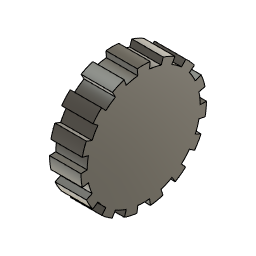
Wheels old (1) (Autodesk Fusion 360 design; units mm, degrees)
Autodesk Fusion 360 part; units mm, degrees
note: some values were not read from the file. Chosen so that the rebuilt part matches the saved one: which face or edge a step refers to.
sketch "Sketch1" plane through (0, 0, 0) normal (1, 0, 0) x (0, 1, 0)
  line L0 (107.0073, 34.7229) -> (118.8971, 38.581)
  line L1 (97.4397, 56.2295) -> (108.2663, 62.4772)
  line L2 (83.5399, 75.3481) -> (92.8221, 83.7201)
  line L3 (66.1554, 90.9929) -> (73.5061, 101.1032)
  line L4 (45.8349, 102.7395) -> (50.9277, 114.155)
  line L5 (0, 112.5) -> (0, 125)
  line L6 (23.3418, 110.0518) -> (25.9354, 122.2798)
  line L7 (0, 112.5) -> (0, 125)
  line L8 (-45.8349, 102.7395) -> (-50.9277, 114.155)
  line L9 (-23.3418, 110.0518) -> (-25.9354, 122.2798)
  line L10 (-66.1554, 90.9929) -> (-73.5061, 101.1032)
  line L11 (-83.5399, 75.3481) -> (-92.8221, 83.7201)
  line L12 (-97.4397, 56.2295) -> (-108.2663, 62.4772)
  line L13 (-107.0073, 34.7229) -> (-118.8971, 38.581)
  line L14 (111.8775, 11.818) -> (124.3084, 13.1312)
  line L15 (-111.8775, 11.818) -> (-124.3084, 13.1312)
  line L16 (111.8775, -11.818) -> (124.3084, -13.1312)
  line L17 (107.0073, -34.7229) -> (118.8971, -38.581)
  line L18 (97.4397, -56.2295) -> (108.2663, -62.4772)
  line L19 (83.5399, -75.3481) -> (92.8221, -83.7201)
  line L20 (66.1554, -90.9929) -> (73.5061, -101.1032)
  line L21 (45.8349, -102.7395) -> (50.9277, -114.155)
  line L22 (23.3418, -110.0518) -> (25.9354, -122.2798)
  line L23 (0, -112.5) -> (0, -125)
  line L24 (-111.8775, -11.818) -> (-124.3084, -13.1312)
  line L25 (-107.0073, -34.7229) -> (-118.8971, -38.581)
  line L26 (-97.4397, -56.2295) -> (-108.2663, -62.4772)
  line L27 (-83.5399, -75.3481) -> (-92.8221, -83.7201)
  line L28 (-66.1554, -90.9929) -> (-73.5061, -101.1032)
  line L29 (-45.8349, -102.7395) -> (-50.9277, -114.155)
  line L30 (-23.3418, -110.0518) -> (-25.9354, -122.2798)
  arc A0 (50.9277, 114.155) -> (25.9354, 122.2798) centre (0, 0) ccw
  arc A1 (92.8221, 83.7201) -> (73.5061, 101.1032) centre (0, 0) ccw
  arc A2 (118.8971, 38.581) -> (108.2663, 62.4772) centre (0, 0) ccw
  arc A3 (124.3084, -13.1312) -> (124.3084, 13.1312) centre (0, 0) ccw
  arc A4 (108.2663, -62.4772) -> (118.8971, -38.581) centre (0, 0) ccw
  arc A5 (73.5061, -101.1032) -> (92.8221, -83.7201) centre (0, 0) ccw
  arc A6 (25.9354, -122.2798) -> (50.9277, -114.155) centre (0, 0) ccw
  arc A7 (-25.9354, -122.2798) -> (0, -125) centre (0, 0) ccw
  arc A8 (-73.5061, -101.1032) -> (-50.9277, -114.155) centre (0, 0) ccw
  arc A9 (-108.2663, -62.4772) -> (-92.8221, -83.7201) centre (0, 0) ccw
  arc A10 (-124.3084, -13.1312) -> (-118.8971, -38.581) centre (0, 0) ccw
  arc A11 (-118.8971, 38.581) -> (-124.3084, 13.1312) centre (0, 0) ccw
  arc A12 (-92.8221, 83.7201) -> (-108.2663, 62.4772) centre (0, 0) ccw
  arc A13 (0, 125) -> (-25.9354, 122.2798) centre (0, 0) ccw
  arc A14 (-50.9277, 114.155) -> (-73.5061, 101.1032) centre (0, 0) ccw
  arc A15 (-23.3418, 110.0518) -> (-45.8349, 102.7395) centre (0, 0) ccw
  arc A16 (-66.1554, 90.9929) -> (-83.5399, 75.3481) centre (0, 0) ccw
  arc A17 (-97.4397, 56.2295) -> (-107.0073, 34.7229) centre (0, 0) ccw
  arc A18 (-111.8775, 11.818) -> (-111.8775, -11.818) centre (0, 0) ccw
  arc A19 (-107.0073, -34.7229) -> (-97.4397, -56.2295) centre (0, 0) ccw
  arc A20 (-83.5399, -75.3481) -> (-66.1554, -90.9929) centre (0, 0) ccw
  arc A21 (-45.8349, -102.7395) -> (-23.3418, -110.0518) centre (0, 0) ccw
  arc A22 (0, -112.5) -> (23.3418, -110.0518) centre (0, 0) ccw
  arc A23 (45.8349, -102.7395) -> (66.1554, -90.9929) centre (0, 0) ccw
  arc A24 (83.5399, -75.3481) -> (97.4397, -56.2295) centre (0, 0) ccw
  arc A25 (107.0073, -34.7229) -> (111.8775, -11.818) centre (0, 0) ccw
  arc A26 (111.8775, 11.818) -> (107.0073, 34.7229) centre (0, 0) ccw
  arc A27 (97.4397, 56.2295) -> (83.5399, 75.3481) centre (0, 0) ccw
  arc A28 (66.1554, 90.9929) -> (45.8349, 102.7395) centre (0, 0) ccw
  arc A29 (23.3418, 110.0518) -> (0, 112.5) centre (0, 0) ccw
  dimension "d3" = 250
  dimension "d4" = 225
  dimension "d5" = 12.4308
  constraint coincident A0.centre A1.centre
  constraint coincident L0.end A13
  constraint coincident L2.end A13
  constraint coincident L4.end A13
  constraint symmetric L0.end L5 L13.end
  constraint symmetric L2.end L5 L11.end
  constraint symmetric L3.end L5 L10.end
  constraint symmetric L4.end L5 L8.end
  constraint coincident L10.start A15
  constraint coincident L11.start A15
  constraint coincident L12.start A15
  constraint coincident L13.start A15
  constraint coincident L15.start A15
  constraint coincident L24.start A15
  constraint coincident L25.start A15
  constraint coincident L27.start A15
  constraint coincident L28.start A15
  constraint coincident L29.start A15
  constraint coincident L30.start A15
  constraint coincident L23.start A15
  constraint coincident L22.start A15
  constraint coincident L21.start A15
  constraint coincident L20.start A15
  constraint coincident L19.start A15
  constraint coincident L18.start A15
  constraint coincident L17.start A15
  constraint coincident L16.start A15
  constraint coincident L14.start A15
  constraint coincident L0.start A15
  constraint coincident L1.start A15
  constraint coincident L2.start A15
  constraint coincident L3.start A15
  constraint coincident L4.start A15
  constraint coincident L6.start A15
  constraint coincident L26.start A15
  constraint coincident L16.end A13
  constraint coincident L18.end A13
  constraint coincident L30.end A13
  constraint coincident L22.end A13
  constraint coincident L26.end A13
  constraint coincident L24.end A13
  constraint concentric A0 A13
  constraint concentric A1 A13
  constraint concentric A2 A13
  constraint concentric A3 A13
  constraint concentric A4 A13
  constraint concentric A5 A13
  constraint concentric A6 A13
  constraint concentric A7 A13
  constraint concentric A8 A13
  constraint concentric A9 A13
  constraint concentric A10 A13
  constraint concentric A11 A13
  constraint concentric A12 A13
  constraint concentric A13 A14
  constraint concentric A15 A16
  constraint concentric A16 A17
  constraint concentric A17 A18
  constraint concentric A18 A19
  constraint concentric A19 A20
  constraint concentric A20 A21
  constraint concentric A21 A22
  constraint concentric A22 A23
  constraint concentric A23 A24
  constraint concentric A24 A25
  constraint concentric A25 A26
  constraint concentric A26 A27
  constraint concentric A27 A28
  constraint concentric A28 A29
  measures "d3" diameter of A13
  measures "d4" diameter of A15
  measures "d5" horizontal distance of L14.start L14.end
extrude "Extrude1" add sketch "Sketch1" along normal blind 20
extrude "Extrude2" cut 1 faces at (0, 4.7652, -44.9254) along direction (1, 0, 0) blind 20
sketch "Sketch4" plane through (0, 0, 0) normal (1, 0, 0) x (0, 1, 0)
sketch "Sketch5" plane through (0, 0, 0) normal (1, 0, 0) x (0, 1, 0)
sketch "Sketch6" plane through (0, 0, 0) normal (1, 0, 0) x (0, 1, 0)
sketch "Sketch7" plane through (0, 0, 0) normal (1, 0, 0) x (0, 1, 0)
sketch "Sketch8" plane through (0, 0, 0) normal (1, 0, 0) x (0, 1, 0)
sketch "Sketch9" plane through (0, 0, 0) normal (1, 0, 0) x (0, 1, 0)
sketch "Sketch10" plane through (0, 0, 0) normal (1, 0, 0) x (0, 1, 0)
sketch "Sketch11" plane through (0, 0, 0) normal (1, 0, 0) x (0, 1, 0)
  circle A0 centre (0, 0) radius 90
  circle A1 centre (0, 0) radius 100
  line L0 (90, 0) -> (99.9996, 0.2793)
  line L1 (90, 0) -> (99.9996, -0.2793)
  line L2 (82.2191, -36.6063) -> (91.2406, -40.9287)
  line L3 (82.2191, -36.6063) -> (91.4678, -40.4183)
  line L4 (27.8115, -85.5951) -> (30.6359, -95.1916)
  line L5 (27.8115, -85.5951) -> (31.1672, -95.019)
  line L6 (60.2218, -66.883) -> (67.1204, -74.1273)
  line L7 (60.2218, -66.883) -> (66.7052, -74.5011)
  line L8 (-88.0333, -18.7121) -> (-97.8725, -20.5179)
  line L9 (-88.0333, -18.7121) -> (-97.7563, -21.0643)
  line L10 (-72.8115, -52.9007) -> (-81.0656, -58.5523)
  line L11 (-72.8115, -52.9007) -> (-80.7372, -59.0043)
  line L12 (-45, -77.9423) -> (-50.2417, -86.4625)
  line L13 (-45, -77.9423) -> (-49.7579, -86.7419)
  line L14 (-9.4076, -89.507) -> (-10.7306, -99.4226)
  line L15 (-9.4076, -89.507) -> (-10.175, -99.481)
  line L16 (-88.0333, 18.7121) -> (-97.8725, 20.5179)
  line L17 (-88.0333, 18.7121) -> (-97.7563, 21.0643)
  line L18 (-72.8115, 52.9007) -> (-81.0656, 58.5523)
  line L19 (-72.8115, 52.9007) -> (-80.7372, 59.0043)
  line L20 (-45, 77.9423) -> (-49.7579, 86.7419)
  line L21 (-45, 77.9423) -> (-50.2417, 86.4625)
  line L22 (-9.4076, 89.507) -> (-10.7306, 99.4226)
  line L23 (-9.4076, 89.507) -> (-10.175, 99.481)
  line L24 (27.8115, 85.5951) -> (30.6359, 95.1916)
  line L25 (27.8115, 85.5951) -> (31.1672, 95.019)
  line L26 (60.2218, 66.883) -> (66.7052, 74.5011)
  line L27 (60.2218, 66.883) -> (67.1204, 74.1273)
  line L28 (82.2191, 36.6063) -> (91.4678, 40.4183)
  line L29 (82.2191, 36.6063) -> (91.2406, 40.9287)
  line L30 (90, 0) -> (99.9996, -0.2793)
  line L31 (90, 0) -> (99.9996, 0.2793)
  line L32 (88.0333, -18.7121) -> (97.8725, -20.5179)
  line L33 (9.4076, 89.507) -> (10.7306, 99.4226)
  line L34 (72.8115, 52.9007) -> (80.7372, 59.0043)
  line L35 (9.4076, 89.507) -> (10.175, 99.481)
  line L36 (45, 77.9423) -> (50.2417, 86.4625)
  line L37 (88.0333, 18.7121) -> (97.8725, 20.5179)
  circle A2 centre (0, 0) radius 100
  line L38 (-90, 0) -> (-99.9996, 0.2793)
  line L39 (9.4076, -89.507) -> (10.175, -99.481)
  line L40 (72.8115, 52.9007) -> (81.0656, 58.5523)
  line L41 (45, 77.9423) -> (49.7579, 86.7419)
  line L42 (-60.2218, -66.883) -> (-66.7052, -74.5011)
  line L43 (-82.2191, -36.6063) -> (-91.4678, -40.4183)
  line L44 (88.0333, 18.7121) -> (97.7563, 21.0643)
  line L45 (45, -77.9423) -> (49.7579, -86.7419)
  circle A3 centre (0, 0) radius 90
  line L46 (72.8115, -52.9007) -> (80.7372, -59.0043)
  line L47 (88.0333, 18.7121) -> (97.7563, 21.0643)
  line L48 (72.8115, -52.9007) -> (81.0656, -58.5523)
  line L49 (45, -77.9423) -> (50.2417, -86.4625)
  line L50 (88.0333, 18.7121) -> (97.8725, 20.5179)
  line L51 (88.0333, -18.7121) -> (97.7563, -21.0643)
  line L52 (-27.8115, 85.5951) -> (-31.1672, 95.019)
  line L53 (9.4076, -89.507) -> (10.7306, -99.4226)
  line L54 (-60.2218, 66.883) -> (-66.7052, 74.5011)
  line L55 (-82.2191, 36.6063) -> (-91.4678, 40.4183)
  line L56 (-27.8115, 85.5951) -> (-30.6359, 95.1916)
  line L57 (-60.2218, -66.883) -> (-67.1204, -74.1273)
  line L58 (-27.8115, -85.5951) -> (-30.6359, -95.1916)
  line L59 (-60.2218, 66.883) -> (-67.1204, 74.1273)
  line L60 (-82.2191, -36.6063) -> (-91.2406, -40.9287)
  line L61 (-27.8115, -85.5951) -> (-31.1672, -95.019)
  line L62 (-82.2191, 36.6063) -> (-91.2406, 40.9287)
  line L63 (-90, 0) -> (-99.9996, -0.2793)
  line L64 (527.8115, 85.5951) -> (530.6359, 95.1916)
  line L65 (410, 0) -> (400.0004, -0.2793)
  line L66 (560.2218, 66.883) -> (566.7052, 74.5011)
  line L67 (582.2191, 36.6063) -> (591.2406, 40.9287)
  line L68 (588.0333, -18.7121) -> (597.7563, -21.0643)
  line L69 (582.2191, 36.6063) -> (591.4678, 40.4183)
  line L70 (588.0333, -18.7121) -> (597.8725, -20.5179)
  line L71 (545, 77.9423) -> (549.7579, 86.7419)
  line L72 (490.5924, 89.507) -> (489.825, 99.481)
  line L73 (411.9667, 18.7121) -> (402.2437, 21.0643)
  line L74 (455, 77.9423) -> (450.2421, 86.7419)
  line L75 (545, -77.9423) -> (549.7579, -86.7419)
  line L76 (527.8115, -85.5951) -> (530.6359, -95.1916)
  line L77 (417.7809, 36.6063) -> (408.5322, 40.4183)
  line L78 (590, 0) -> (599.9996, 0.2793)
  line L79 (545, -77.9423) -> (550.2417, -86.4625)
  line L80 (590, 0) -> (599.9996, -0.2793)
  line L81 (417.7809, 36.6063) -> (408.7594, 40.9287)
  line L82 (590, 0) -> (599.9996, -0.2793)
  line L83 (411.9667, 18.7121) -> (402.1275, 20.5179)
  line L84 (588.0333, 18.7121) -> (597.7563, 21.0643)
  line L85 (527.8115, 85.5951) -> (531.1672, 95.019)
  line L86 (545, 77.9423) -> (550.2417, 86.4625)
  line L87 (509.4076, 89.507) -> (510.7306, 99.4226)
  line L88 (572.8115, 52.9007) -> (580.7372, 59.0043)
  line L89 (560.2218, 66.883) -> (567.1204, 74.1273)
  line L90 (588.0333, 18.7121) -> (597.7563, 21.0643)
  line L91 (582.2191, -36.6063) -> (591.4678, -40.4183)
  line L92 (427.1885, 52.9007) -> (419.2628, 59.0043)
  line L93 (439.7782, 66.883) -> (433.2948, 74.5011)
  line L94 (572.8115, -52.9007) -> (581.0656, -58.5523)
  line L95 (417.7809, -36.6063) -> (408.7594, -40.9287)
  line L96 (472.1885, 85.5951) -> (468.8328, 95.019)
  line L97 (560.2218, -66.883) -> (567.1204, -74.1273)
  line L98 (590, 0) -> (599.9996, 0.2793)
  line L99 (527.8115, -85.5951) -> (531.1672, -95.019)
  line L100 (509.4076, -89.507) -> (510.175, -99.481)
  line L101 (427.1885, -52.9007) -> (419.2628, -59.0043)
  line L102 (472.1885, -85.5951) -> (469.3641, -95.1916)
  line L103 (582.2191, -36.6063) -> (591.2406, -40.9287)
  line L104 (490.5924, -89.507) -> (489.2694, -99.4226)
  line L105 (509.4076, -89.507) -> (510.7306, -99.4226)
  line L106 (490.5924, 89.507) -> (489.2694, 99.4226)
  line L107 (472.1885, -85.5951) -> (468.8328, -95.019)
  line L108 (439.7782, 66.883) -> (432.8796, 74.1273)
  line L109 (572.8115, -52.9007) -> (580.7372, -59.0043)
  line L110 (472.1885, 85.5951) -> (469.3641, 95.1916)
  line L111 (455, 77.9423) -> (449.7583, 86.4625)
  line L112 (572.8115, 52.9007) -> (581.0656, 58.5523)
  line L113 (560.2218, -66.883) -> (566.7052, -74.5011)
  line L114 (410, 0) -> (400.0004, 0.2793)
  line L115 (455, -77.9423) -> (449.7583, -86.4625)
  line L116 (439.7782, -66.883) -> (432.8796, -74.1273)
  line L117 (417.7809, -36.6063) -> (408.5322, -40.4183)
  line L118 (455, -77.9423) -> (450.2421, -86.7419)
  line L119 (509.4076, 89.507) -> (510.175, 99.481)
  line L120 (411.9667, -18.7121) -> (402.1275, -20.5179)
  line L121 (427.1885, 52.9007) -> (418.9344, 58.5523)
  line L122 (490.5924, -89.507) -> (489.825, -99.481)
  line L123 (411.9667, -18.7121) -> (402.2437, -21.0643)
  line L124 (427.1885, -52.9007) -> (418.9344, -58.5523)
  line L125 (439.7782, -66.883) -> (433.2948, -74.5011)
  line L126 (0, 900) -> (500, 900)
  line L127 (0, 900) -> (0, 800)
  arc A4 (0, 900) -> (0, 700) centre (0, 800) ccw
  line L128 (0, 700) -> (500, 700)
  arc A5 (500, 700) -> (500, 900) centre (500, 800) ccw
  line L129 (0, 800) -> (0, 890)
  line L130 (0, 890) -> (500, 890)
  line L131 (500, 890) -> (500, 800)
  line L132 (500, 800) -> (500, 710)
  line L133 (500, 710) -> (0, 710)
  line L134 (0, 710) -> (0, 800)
  arc A6 (0, 890) -> (0, 710) centre (0, 800) ccw
  arc A7 (500, 710) -> (500, 890) centre (500, 800) ccw
  line L135 (472.1885, 85.5951) -> (472.001, 86.1215)
  line L136 (472.1885, 85.5951) -> (472.001, 86.1215)
  line L137 (500, 0) -> (600, 0) construction
  arc A8 (588.0333, 18.7121) -> (509.4076, 89.507) centre (500, 0) ccw
  line L138 (598.7688, 15.6434) -> (588.8478, 14.3549)
  line L139 (599.863, 5.2336) -> (589.8908, 4.4313)
  arc A9 (490.5924, 89.507) -> (590, 0) centre (500, 0) ccw
  arc A10 (589.8908, 4.4313) -> (588.8478, 14.3549) centre (500, 0) ccw
  arc A11 (588.0333, 18.7121) -> (590, 0) centre (500, 0) ccw
  arc A12 (589.8908, 4.4313) -> (588.892, 14.0791) centre (500, 0) ccw
  arc A13 (597.7563, 21.0643) -> (599.9996, 0.2793) centre (500, 0) ccw
  arc A14 (599.863, 5.2336) -> (598.7688, 15.6434) centre (500, 0) ccw
  arc A15 (597.7563, 21.0643) -> (599.9996, 0.2793) centre (500, 0) ccw
  arc A16 (599.863, 5.2336) -> (598.7688, 15.6434) centre (500, 0) ccw
  line L140 (538.8307, 157.1135) -> (539.0166, 147.1109)
  arc A17 (549.2978, 157.0522) -> (538.8307, 157.1135) centre (543.4794, 57.2216) ccw
  arc A18 (548.9948, 147.0525) -> (539.0166, 147.1109) centre (543.4794, 57.2216) ccw
  line L141 (549.2978, 157.0522) -> (548.9948, 147.0525)
  arc A19 (548.9948, 147.0525) -> (539.2956, 147.1243) centre (543.4794, 57.2216) ccw
  arc A20 (549.2978, 157.0522) -> (538.8307, 157.1135) centre (543.4794, 57.2216) ccw
  line L142 (500, 0) -> (503.1052, 0)
  line L143 (500, 0) -> (503.1052, 0)
  dimension "d41" = 180
  dimension "d42" = 200
  dimension "d58" = 180
  dimension "d59" = 200
  constraint coincident A0.centre A1.centre
  constraint coincident A1 L0.end
  constraint coincident A1 L1.end
  constraint coincident A1 L3.end
  constraint coincident A1 L2.end
  constraint coincident A1 L7.end
  constraint coincident A1 L6.end
  constraint coincident A1 L4.end
  constraint coincident A1 L5.end
  constraint coincident A1 L15.end
  constraint coincident A1 L14.end
  constraint coincident A1 L12.end
  constraint coincident A1 L13.end
  constraint coincident A1 L10.end
  constraint coincident A1 L11.end
  constraint coincident A1 L8.end
  constraint coincident A1 L9.end
  constraint coincident A1 L17.end
  constraint coincident A1 L16.end
  constraint coincident A1 L18.end
  constraint coincident A1 L19.end
  constraint coincident A1 L21.end
  constraint coincident A1 L20.end
  constraint coincident A1 L23.end
  constraint coincident A1 L22.end
  constraint coincident A1 L24.end
  constraint coincident A1 L25.end
  constraint coincident A1 L27.end
  constraint coincident A1 L26.end
  constraint coincident A1 L29.end
  constraint coincident A1 L28.end
  constraint coincident L80.end A13
  constraint coincident L91.end A13
  constraint coincident L103.end A13
  constraint coincident L113.end A13
  constraint coincident L97.end A13
  constraint coincident L76.end A13
  constraint coincident L99.end A13
  constraint coincident L122.end A13
  constraint coincident L104.end A13
  constraint coincident L115.end A13
  constraint coincident L118.end A13
  constraint coincident L124.end A13
  constraint coincident L101.end A13
  constraint coincident L120.end A13
  constraint coincident L123.end A13
  constraint coincident L73.end A13
  constraint coincident L83.end A13
  constraint coincident L121.end A13
  constraint coincident L92.end A13
  constraint coincident L111.end A13
  constraint coincident L74.end A13
  constraint coincident L72.end A13
  constraint coincident L106.end A13
  constraint coincident L64.end A13
  constraint coincident L85.end A13
  constraint coincident L89.end A13
  constraint coincident L66.end A13
  constraint coincident L67.end A13
  constraint coincident L69.end A13
  constraint horizontal L126
  constraint perpendicular L126 L127
  constraint coincident L127.end A4.centre
  constraint tangent A4 L128
  constraint horizontal L128
  constraint coincident L127 L129.end
  constraint parallel L127 L129
  constraint perpendicular L129 L130
  constraint coincident A5.centre L131.end
  constraint perpendicular L130 L131
  constraint perpendicular L130 L132
  constraint perpendicular L131 L133
  constraint perpendicular L133 L134
  constraint coincident L132 L133.start
  constraint coincident L96 L135.end
  constraint parallel L96 L136
  constraint horizontal L137
  constraint coincident L137.start A8.centre
  constraint concentric A8 A9
  constraint coincident L139.end A11
  constraint concentric A9 A10
  constraint concentric A11 A12
  constraint concentric A13 A14
  constraint concentric A15 A16
  constraint parallel L142 L143
  measures "d41" diameter of A0
  measures "d42" diameter of A1
  measures "d58" diameter of A11
  measures "d59" diameter of A13
extrude "Extrude4" add sketch "Sketch11" along normal blind 50 contours A0 A3 | A0 A1 L1 L30 L32 A2 A3 | A0 A1 L28 A2 L44 A3 L47 | A0 A1 L2 A2 A3 L48 | A0 A1 L27 L34 A2 A3 | A0 A1 L7 A2 A3 L49 | A0 A1 L25 A2 L41 A3 | A0 A1 L4 A2 A3 L53 | A0 A1 L23 L35 A2 A3 | A0 A1 L14 A2 A3 L58 | A0 A1 L20 A2 A3 L52 | A0 A1 L12 A2 L42 A3 | A0 A1 L19 A2 A3 L59 | A0 A1 L10 A2 A3 L60 | A0 A1 L17 A2 A3 L55 | A0 A1 L8 A2 A3 L63
extrude "Extrude3" [suppressed]
sketch "Sketch12" plane through (50, 0, 0) normal (1, 0, 0) x (0, 1, 0)
  arc A0 (-88.0333, 18.7121) -> (-90, 0) centre (0, 0) ccw
  line L0 (-90, 0) -> (-99.9996, -0.2793)
  arc A1 (-99.9996, -0.2793) -> (-97.8725, -20.5179) centre (0, 0) ccw
  line L1 (-97.8725, -20.5179) -> (-88.0333, -18.7121)
  arc A2 (-88.0333, -18.7121) -> (-82.2191, -36.6063) centre (0, 0) ccw
  line L2 (-82.2191, -36.6063) -> (-91.2406, -40.9287)
  arc A3 (-91.2406, -40.9287) -> (-81.0656, -58.5523) centre (0, 0) ccw
  line L3 (-81.0656, -58.5523) -> (-72.8115, -52.9007)
  arc A4 (-72.8115, -52.9007) -> (-60.2218, -66.883) centre (0, 0) ccw
  line L4 (-60.2218, -66.883) -> (-66.7052, -74.5011)
  arc A5 (-66.7052, -74.5011) -> (-50.2417, -86.4625) centre (0, 0) ccw
  line L5 (-50.2417, -86.4625) -> (-45, -77.9423)
  arc A6 (-45, -77.9423) -> (-27.8115, -85.5951) centre (0, 0) ccw
  line L6 (-27.8115, -85.5951) -> (-30.6359, -95.1916)
  arc A7 (-30.6359, -95.1916) -> (-10.7306, -99.4226) centre (0, 0) ccw
  line L7 (-10.7306, -99.4226) -> (-9.4076, -89.507)
  arc A8 (-9.4076, -89.507) -> (9.4076, -89.507) centre (0, 0) ccw
  line L8 (9.4076, -89.507) -> (10.7306, -99.4226)
  arc A9 (10.7306, -99.4226) -> (30.6359, -95.1916) centre (0, 0) ccw
  line L9 (30.6359, -95.1916) -> (27.8115, -85.5951)
  arc A10 (27.8115, -85.5951) -> (45, -77.9423) centre (0, 0) ccw
  line L10 (45, -77.9423) -> (50.2417, -86.4625)
  arc A11 (50.2417, -86.4625) -> (66.7052, -74.5011) centre (0, 0) ccw
  line L11 (66.7052, -74.5011) -> (60.2218, -66.883)
  arc A12 (60.2218, -66.883) -> (72.8115, -52.9007) centre (0, 0) ccw
  line L12 (72.8115, -52.9007) -> (81.0656, -58.5523)
  arc A13 (81.0656, -58.5523) -> (91.2406, -40.9287) centre (0, 0) ccw
  line L13 (91.2406, -40.9287) -> (82.2191, -36.6063)
  arc A14 (82.2191, -36.6063) -> (88.0333, -18.7121) centre (0, 0) ccw
  line L14 (88.0333, -18.7121) -> (97.8725, -20.5179)
  arc A15 (97.8725, -20.5179) -> (99.9996, -0.2793) centre (0, 0) ccw
  line L15 (99.9996, -0.2793) -> (90, 0)
  arc A16 (90, 0) -> (88.0333, 18.7121) centre (0, 0) ccw
  line L16 (88.0333, 18.7121) -> (97.7563, 21.0643)
  arc A17 (97.7563, 21.0643) -> (91.4678, 40.4183) centre (0, 0) ccw
  line L17 (91.4678, 40.4183) -> (82.2191, 36.6063)
  arc A18 (82.2191, 36.6063) -> (72.8115, 52.9007) centre (0, 0) ccw
  line L18 (72.8115, 52.9007) -> (80.7372, 59.0043)
  arc A19 (80.7372, 59.0043) -> (67.1204, 74.1273) centre (0, 0) ccw
  line L19 (67.1204, 74.1273) -> (60.2218, 66.883)
  arc A20 (60.2218, 66.883) -> (45, 77.9423) centre (0, 0) ccw
  line L20 (45, 77.9423) -> (49.7579, 86.7419)
  arc A21 (49.7579, 86.7419) -> (31.1672, 95.019) centre (0, 0) ccw
  line L21 (31.1672, 95.019) -> (27.8115, 85.5951)
  arc A22 (27.8115, 85.5951) -> (9.4076, 89.507) centre (0, 0) ccw
  line L22 (9.4076, 89.507) -> (10.175, 99.481)
  arc A23 (10.175, 99.481) -> (-10.175, 99.481) centre (0, 0) ccw
  line L23 (-10.175, 99.481) -> (-9.4076, 89.507)
  arc A24 (-9.4076, 89.507) -> (-27.8115, 85.5951) centre (0, 0) ccw
  line L24 (-27.8115, 85.5951) -> (-31.1672, 95.019)
  arc A25 (-31.1672, 95.019) -> (-49.7579, 86.7419) centre (0, 0) ccw
  line L25 (-49.7579, 86.7419) -> (-45, 77.9423)
  arc A26 (-45, 77.9423) -> (-60.2218, 66.883) centre (0, 0) ccw
  line L26 (-60.2218, 66.883) -> (-67.1204, 74.1273)
  arc A27 (-67.1204, 74.1273) -> (-80.7372, 59.0043) centre (0, 0) ccw
  line L27 (-80.7372, 59.0043) -> (-72.8115, 52.9007)
  arc A28 (-72.8115, 52.9007) -> (-82.2191, 36.6063) centre (0, 0) ccw
  line L28 (-82.2191, 36.6063) -> (-91.4678, 40.4183)
  arc A29 (-91.4678, 40.4183) -> (-97.7563, 21.0643) centre (0, 0) ccw
  line L29 (-97.7563, 21.0643) -> (-88.0333, 18.7121)
sketch "Sketch13" plane through (0, 0, 0) normal (1, 0, 0) x (0, 1, 0)
sketch "Sketch2" plane through (20, 0, 0) normal (1, 0, 0) x (0, 1, 0)
  arc A0 (66.1554, 90.9929) -> (45.8349, 102.7395) centre (0, 0) ccw
  line L0 (45.8349, 102.7395) -> (50.9277, 114.155)
  arc A1 (50.9277, 114.155) -> (25.9354, 122.2798) centre (0, 0) ccw
  line L1 (25.9354, 122.2798) -> (23.3418, 110.0518)
  arc A2 (23.3418, 110.0518) -> (0, 112.5) centre (0, 0) ccw
  line L2 (0, 112.5) -> (0, 125)
  arc A3 (0, 125) -> (-25.9354, 122.2798) centre (0, 0) ccw
  line L3 (-25.9354, 122.2798) -> (-23.3418, 110.0518)
  arc A4 (-23.3418, 110.0518) -> (-45.8349, 102.7395) centre (0, 0) ccw
  line L4 (-45.8349, 102.7395) -> (-50.9277, 114.155)
  arc A5 (-50.9277, 114.155) -> (-73.5061, 101.1032) centre (0, 0) ccw
  line L5 (-73.5061, 101.1032) -> (-66.1554, 90.9929)
  arc A6 (-66.1554, 90.9929) -> (-83.5399, 75.3481) centre (0, 0) ccw
  line L6 (-83.5399, 75.3481) -> (-92.8221, 83.7201)
  arc A7 (-92.8221, 83.7201) -> (-108.2663, 62.4772) centre (0, 0) ccw
  line L7 (-108.2663, 62.4772) -> (-97.4397, 56.2295)
  arc A8 (-97.4397, 56.2295) -> (-107.0073, 34.7229) centre (0, 0) ccw
  line L8 (-107.0073, 34.7229) -> (-118.8971, 38.581)
  arc A9 (-118.8971, 38.581) -> (-124.3084, 13.1312) centre (0, 0) ccw
  line L9 (-124.3084, 13.1312) -> (-111.8775, 11.818)
  arc A10 (-111.8775, 11.818) -> (-111.8775, -11.818) centre (0, 0) ccw
  line L10 (-111.8775, -11.818) -> (-124.3084, -13.1312)
  arc A11 (-124.3084, -13.1312) -> (-118.8971, -38.581) centre (0, 0) ccw
  line L11 (-118.8971, -38.581) -> (-107.0073, -34.7229)
  arc A12 (-107.0073, -34.7229) -> (-97.4397, -56.2295) centre (0, 0) ccw
  line L12 (-97.4397, -56.2295) -> (-108.2663, -62.4772)
  arc A13 (-108.2663, -62.4772) -> (-92.8221, -83.7201) centre (0, 0) ccw
  line L13 (-92.8221, -83.7201) -> (-83.5399, -75.3481)
  arc A14 (-83.5399, -75.3481) -> (-66.1554, -90.9929) centre (0, 0) ccw
  line L14 (-66.1554, -90.9929) -> (-73.5061, -101.1032)
  arc A15 (-73.5061, -101.1032) -> (-50.9277, -114.155) centre (0, 0) ccw
  line L15 (-50.9277, -114.155) -> (-45.8349, -102.7395)
  arc A16 (-45.8349, -102.7395) -> (-23.3418, -110.0518) centre (0, 0) ccw
  line L16 (-23.3418, -110.0518) -> (-25.9354, -122.2798)
  arc A17 (-25.9354, -122.2798) -> (0, -125) centre (0, 0) ccw
  line L17 (0, -125) -> (0, -112.5)
  arc A18 (0, -112.5) -> (23.3418, -110.0518) centre (0, 0) ccw
  line L18 (23.3418, -110.0518) -> (25.9354, -122.2798)
  arc A19 (25.9354, -122.2798) -> (50.9277, -114.155) centre (0, 0) ccw
  line L19 (50.9277, -114.155) -> (45.8349, -102.7395)
  arc A20 (45.8349, -102.7395) -> (66.1554, -90.9929) centre (0, 0) ccw
  line L20 (66.1554, -90.9929) -> (73.5061, -101.1032)
  arc A21 (73.5061, -101.1032) -> (92.8221, -83.7201) centre (0, 0) ccw
  line L21 (92.8221, -83.7201) -> (83.5399, -75.3481)
  arc A22 (83.5399, -75.3481) -> (97.4397, -56.2295) centre (0, 0) ccw
  line L22 (97.4397, -56.2295) -> (108.2663, -62.4772)
  arc A23 (108.2663, -62.4772) -> (118.8971, -38.581) centre (0, 0) ccw
  line L23 (118.8971, -38.581) -> (107.0073, -34.7229)
  arc A24 (107.0073, -34.7229) -> (111.8775, -11.818) centre (0, 0) ccw
  line L24 (111.8775, -11.818) -> (124.3084, -13.1312)
  arc A25 (124.3084, -13.1312) -> (124.3084, 13.1312) centre (0, 0) ccw
  line L25 (124.3084, 13.1312) -> (111.8775, 11.818)
  arc A26 (111.8775, 11.818) -> (107.0073, 34.7229) centre (0, 0) ccw
  line L26 (107.0073, 34.7229) -> (118.8971, 38.581)
  arc A27 (118.8971, 38.581) -> (108.2663, 62.4772) centre (0, 0) ccw
  line L27 (108.2663, 62.4772) -> (97.4397, 56.2295)
  arc A28 (97.4397, 56.2295) -> (83.5399, 75.3481) centre (0, 0) ccw
  line L28 (83.5399, 75.3481) -> (92.8221, 83.7201)
  arc A29 (92.8221, 83.7201) -> (73.5061, 101.1032) centre (0, 0) ccw
  line L29 (73.5061, 101.1032) -> (66.1554, 90.9929)
sketch "Sketch3" plane through (20, 0.6935, 0) normal (1, 0, 0) x (0, 1, 0)
